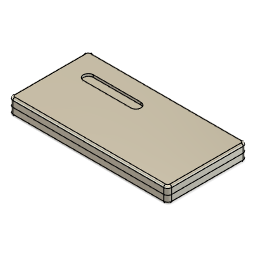
Breadboard Box v1 (Autodesk Fusion 360 design; units mm, degrees)
Autodesk Fusion 360 part; units mm, degrees
sketch "Sketch2" plane through (0, 0, 0) normal (0, 1, 0) x (1, 0, 0)
  line L0 (100, 50) -> (-100, 50)
  line L1 (-100, 50) -> (-100, -50)
  line L2 (-100, -50) -> (100, -50)
  line L3 (100, -50) -> (100, 50)
  line L4 (100, 50) -> (-100, -50) construction
  line L5 (-100, 50) -> (100, -50) construction
  dimension "d1" = 100
  dimension "d2" = 200
  constraint perpendicular L0 L1
  constraint parallel L0 L2
  constraint parallel L1 L3
  constraint horizontal L0
  constraint coincident L4 origin
  constraint coincident L5 origin
  measures "d1" distance of L0 L2
  measures "d2" distance of L1 L3
extrude "Extrude1" add sketch "Sketch2" along normal blind 20 makes body 1
fillet "Fillet1" radius 5 4 edges at (100, 10, -50) (100, 10, 50) (-100, 10, 50) (-100, 10, -50) on bodies 1
fillet "Fillet2" radius 2.5 16 edges at (98.5355, 20, -48.5355) (0, 20, -50) (-98.5355, 20, -48.5355) (-100, 20, 0) (-98.5355, 20, 48.5355) (0, 20, 50) (98.5355, 20, 48.5355) (100, 20, 0) (0, 0, -50) (-98.5355, 0, -48.5355) (-100, 0, 0) (-98.5355, 0, 48.5355) (0, 0, 50) (98.5355, 0, 48.5355) (100, 0, 0) (98.5355, 0, -48.5355) on bodies 1
ref_plane "WorkPlane1" through (0, 10, 0) normal (0, 1, 0) x (0, 0, 1)
shell "Shell2" thickness 3 removed faces 0 bodies 1
split "Split1" by plane through (0, 10, 0) normal (0, 1, 0) bodies 1 makes body 2 at (31.6667, 20, 15.8333)
sketch "Sketch3" plane through (0, 10, 0) normal (0, 1, 0) x (-1, 0, 0)
  line L0 (100, -45) -> (100, 45)
  arc A0 (100, 45) -> (95, 50) centre (95, 45) ccw
  line L1 (95, 50) -> (-95, 50)
  arc A1 (-95, 50) -> (-100, 45) centre (-95, 45) ccw
  line L2 (-100, 45) -> (-100, -45)
  arc A2 (-100, -45) -> (-95, -50) centre (-95, -45) ccw
  line L3 (-95, -50) -> (95, -50)
  arc A3 (95, -50) -> (100, -45) centre (95, -45) ccw
  arc A4 (97, 45) -> (95, 47) centre (95, 45) ccw
  line L4 (97, 45) -> (97, -45)
  arc A5 (95, -47) -> (97, -45) centre (95, -45) ccw
  line L5 (95, -47) -> (-95, -47)
  arc A6 (-97, -45) -> (-95, -47) centre (-95, -45) ccw
  line L6 (-97, -45) -> (-97, 45)
  arc A7 (-95, 47) -> (-97, 45) centre (-95, 45) ccw
  line L7 (-95, 47) -> (95, 47)
  line L8 (99, -45) -> (99, 45)
  arc A8 (99, 45) -> (95, 49) centre (95, 45) ccw
  line L9 (95, 49) -> (-95, 49)
  arc A9 (-95, 49) -> (-99, 45) centre (-95, 45) ccw
  line L10 (-99, 45) -> (-99, -45)
  arc A10 (-99, -45) -> (-95, -49) centre (-95, -45) ccw
  line L11 (-95, -49) -> (95, -49)
  arc A11 (95, -49) -> (99, -45) centre (95, -45) ccw
  line L12 (98, -45) -> (98, 45)
  arc A12 (98, 45) -> (95, 48) centre (95, 45) ccw
  line L13 (95, 48) -> (-95, 48)
  arc A13 (-95, 48) -> (-98, 45) centre (-95, 45) ccw
  line L14 (-98, 45) -> (-98, -45)
  arc A14 (-98, -45) -> (-95, -48) centre (-95, -45) ccw
  line L15 (-95, -48) -> (95, -48)
  arc A15 (95, -48) -> (98, -45) centre (95, -45) ccw
  dimension "d9" = -1
  dimension "d10" = -2
extrude "Extrude2" add sketch "Sketch3" along normal blind 1 contours L8 A8 L9 A9 L10 A10 L11 A11 bodies 1
fillet "Fillet3" radius 0.25 16 edges at (-97.8284, 11, -47.8284) (-99, 11, 0) (-97.8284, 11, 47.8284) (0, 11, 49) (97.8284, 11, 47.8284) (99, 11, 0) (97.8284, 11, -47.8284) (0, 11, -49) (98, 11, 0) (97.1213, 11, 47.1213) (0, 11, 48) (-97.1213, 11, 47.1213) (-98, 11, 0) (-97.1213, 11, -47.1213) (0, 11, -48) (97.1213, 11, -47.1213) on bodies 1
combine "Combine1" operation cut target body 2 tool bodies 1 keep tools
sketch "Sketch4" plane through (0, 20, 0) normal (0, 1, 0) x (-1, 0, 0)
  arc A0 (-97.5, -45) -> (-95, -47.5) centre (-95, -45) ccw
  line L0 (-95, -47.5) -> (95, -47.5)
  arc A1 (95, -47.5) -> (97.5, -45) centre (95, -45) ccw
  line L1 (97.5, -45) -> (97.5, 45)
  arc A2 (97.5, 45) -> (95, 47.5) centre (95, 45) ccw
  line L2 (95, 47.5) -> (-95, 47.5)
  arc A3 (-95, 47.5) -> (-97.5, 45) centre (-95, 45) ccw
  line L3 (-97.5, 45) -> (-97.5, -45)
  line L4 (70, -13.7265) -> (10, -13.7265)
  arc A4 (10, -13.7265) -> (10, -26.2735) centre (10, -20) ccw
  line L5 (10, -26.2735) -> (70, -26.2735)
  arc A5 (70, -26.2735) -> (70, -13.7265) centre (70, -20) ccw
  line L6 (70, -20) -> (10, -20) construction
  constraint tangent L4 A4
  constraint tangent A4 L5
  constraint parallel L4 L5
  constraint tangent L5 A5
  constraint tangent L4 A5
  constraint horizontal L6
extrude "Extrude3" cut sketch "Sketch4" against normal up to surface (3 mm away) contours L4 A4 L5 A5 bodies 2
named bodies: "Bottom", "Top"
